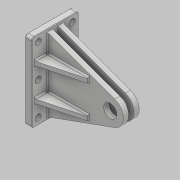
# Autodesk Inventor part: exercise3-19ipt
Saved by Autodesk Inventor 2018 (Build 220112000, 112)
## iProperties
Created: 2020-09-23
Part Number: exercise3-19ipt
Material: 一般
Document SubType Name: Modeling
Designer: 王鼎鈞
Density: 1 g/cm^3
Appearance: 預設
Author: 王鼎鈞
Autodesk Inventor part; units mm, degrees
sketch "草圖1" plane through (0, 0, 0) normal (1, 0, 0) x (0, 1, 0)
  line L0 (-90, 150) -> (90, 150)
  line L1 (90, 150) -> (90, -150)
  line L2 (90, -150) -> (-90, -150)
  line L3 (-90, -150) -> (-90, 150)
  line L4 (-90, 150) -> (90, -150) construction
  line L5 (90, 150) -> (-90, -150) construction
  point P0 (0, 0)
  dimension "d0" = 180
  dimension "d1" = 300
  constraints: 12 end point, 2 midpoint, 2 parallel, 1 horizontal, 1 perpendicular
  measures "d0" distance of L1.end L2.end
  measures "d1" distance of L0.end L1.end
extrude "擠出1" add sketch "草圖1" along normal blind 25
fillet "圓角1" radius 10 4 edges at (12.5, 90, 150) (12.5, -90, 150) (12.5, 90, -150) (12.5, -90, -150)
chamfer "倒角1" distance 2 angle 45 16 edges at (25, 90, 0) (25, 87.0711, 147.0711) (25, 0, 150) (25, -87.0711, 147.0711) (25, -90, 0) (25, -87.0711, -147.0711) (25, 0, -150) (25, 87.0711, -147.0711) (0, 90, 0) (0, 87.0711, -147.0711) (0, 0, -150) (0, -87.0711, -147.0711) (0, -90, 0) (0, -87.0711, 147.0711) (0, 0, 150) (0, 87.0711, 147.0711)
sketch "草圖2" plane through (25, 0, 0) normal (1, 0, 0) x (0, 0, -1)
  line L0 (-150, 80) -> (-150, -80) projected
  line L1 (0, -126) -> (0, 126) projected
  line L2 (210, 0) -> (-210, 0) projected
  line L3 (-125, -126) -> (-125, 126)
  line L4 (210, 65) -> (-210, 65)
  point P0 (0, 0)
  point P1 (-125, 65)
  dimension "d8" = 125
  dimension "d9" = 65
  constraints: 4 end point, 2 parallel, 2 point on line
  measures "d8" distance between parallel lines of L1 L3
  measures "d9" distance between parallel lines of L2 L4
hole "孔1" at (25, 65, 125) direction (-1, 0, 0) diameter 20 end through all
chamfer "倒角2" distance 2 angle 45 2 edges at (25, 65, 135) (0, 65, 135)
pattern_linear "矩形陣列1" count 3 spacing 125 along (0, 0, -1) of "孔1", "倒角2"
ref_plane "工作平面1" through (2, 0, -140) normal (0, -1, 0) x (1, 0, 0)
mirror "鏡射1" about plane through (2, 0, -140) normal (0, -1, 0) of "孔1", "倒角2", "矩形陣列1"
ref_plane "工作平面3" through (2, 10, -140) normal (0, -1, 0) x (1, 0, 0)
ref_plane "工作平面2" through (2, 0, -140) normal (0, -1, 0) x (1, 0, 0)
sketch "草圖3" plane through (2, 10, -140) normal (0, -1, 0) x (1, 0, 0)
  line L0 (-65, 140) -> (376, 140) projected
  line L1 (-2, -70) -> (-2, 350) projected
  circle A0 centre (263, 140) radius 25
  arc A1 (280.0102, 92.9824) -> (280.0102, 187.0176) centre (263, 140) ccw
  line L2 (23, 280) -> (23, 0) projected
  line L3 (23, 140) -> (23, 280)
  line L4 (23, 280) -> (280.0102, 187.0176)
  line L5 (23, 140) -> (23, 0)
  line L6 (23, 128) -> (23, 152) projected
  line L7 (23, 0) -> (280.0102, 92.9824)
  point P0 (-2, 140)
  dimension "d24" = 50
  dimension "d25" = 100
  dimension "d26" = 240
  dimension "d27" = 140
  dimension "d28" = 140
  constraints: 8 end point, 2 centre point, 2 collinear, 2 point on circle, 2 tangent, 1 coincident, 1 midpoint, 1 point on line
  measures "d24" diameter of A0
  measures "d25" diameter of A1
  measures "d26" distance from line of L2 A1.centre
  measures "d27" distance of L3.start L2.start
  measures "d28" distance of L3.start L2.end
extrude "擠出2" add sketch "草圖3" against normal blind 20 contours L2 L4 A1 L0 A0 | L0 A0 A1 L7 L2
ref_plane "工作平面5" through (-325.7492, 65, 55) normal (0, 0, 1) x (1, 0, 0)
ref_plane "工作平面4" through (-325.7492, 65, 0) normal (0, 0, 1) x (1, 0, 0)
sketch "草圖4" plane through (-325.7492, 65, 55) normal (0, 0, 1) x (1, 0, 0)
  line L0 (350.7492, 15) -> (350.7492, -145) projected
  line L1 (350.7492, -35) -> (350.7492, 15)
  line L2 (350.7492, 15) -> (510.7492, -27.8719)
  line L3 (510.7492, -27.8719) -> (510.7492, -35)
  line L4 (510.7492, -35) -> (510.7492, -35)
  line L5 (607.7594, -35) -> (350.7492, -35) projected
  line L6 (510.7492, -35) -> (350.7492, -35)
  line L7 (350.7492, -35) -> (350.7492, -25)
  line L8 (350.7492, -25) -> (360.7492, -35)
  point P0 (325.7492, -65)
  dimension "d34" = 50
  dimension "d35" = 75
  dimension "d36" = 160
  dimension "d37" = 0
  dimension "d38" = 10
  dimension "d39" = 45
  constraints: 14 end point, 5 point on line, 2 vertical, 1 perpendicular
  measures "d34" distance of L1.start L1.end
  measures "d35" angle of L0 L2
  measures "d36" distance from line of L0 L2.end
  measures "d37" distance from line of L1.start L5
  measures "d38" distance of L5.end L7.end
  measures "d39" angle of L7 L8
extrude "擠出3" add sketch "草圖4" along normal blind 15 contours L2 L3 L5 L8 L0
mirror "鏡射2" about plane through (-325.7492, 65, 0) normal (0, 0, 1) of "擠出3"
mirror "鏡射3" about plane through (2, 0, -140) normal (0, -1, 0) of "擠出3", "鏡射2", "擠出2"
chamfer "倒角3" distance 5 angle 45 18 edges at (110, 30, -55) (25, 60, -55) (25, 30, 0) (25, 60, -70) (110, 30, -70) (110, 30, 55) (110, 30, 70) (25, 60, 70) (25, 60, 55) (25, -60, 70) (25, -30, 0) (110, -30, 70) (110, -30, 55) (25, -60, 55) (110, -30, -55) (25, -60, -55) (110, -30, -70) (25, -60, -70)
